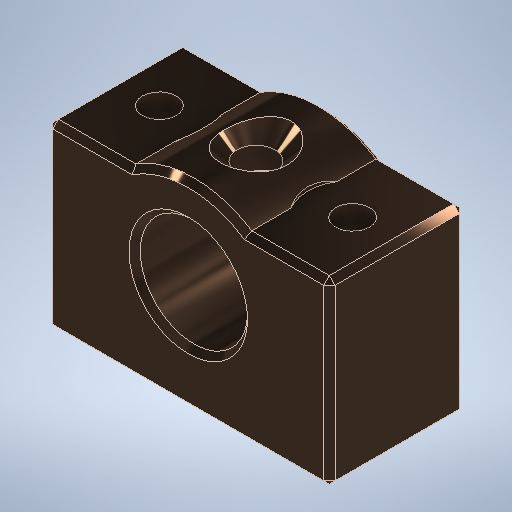
# Autodesk Inventor part: 05 Crankbearing
Saved by Autodesk Inventor 2025.2 (Build 292293000, 293)
## iProperties
Created: 2025-07-30
Part Number: 05 Crankbearing
Material: Bronze
Document SubType Name: Modeling
Designer: bless
Density: 8.47 g/cm^3
Appearance: Bronze - Polished
Author: bless
Autodesk Inventor part; units mm, degrees
ref_plane "YZ Plane" through (0, 0, 0) normal (1, 0, 0) x (0, 1, 0)
ref_plane "XY Plane" through (0, 0, 0) normal (0, 0, 1) x (1, 0, 0)
sketch "Sketch1" plane through (0, 0, 0) normal (0, 0, 1) x (1, 0, 0)
  line L0 (0, 0) -> (25, 0)
  line L1 (25, 0) -> (25, 16)
  line L2 (25, 16) -> (0, 16)
  line L3 (0, 16) -> (0, 0)
  circle A0 centre (12.5, 9.5) radius 4.75
  arc A1 (17.6235, 16) -> (7.3765, 16) centre (12.5, 8) ccw
  point P0 (12.5, 16)
  point P1 (0, 8)
  dimension "d0" = 25
  dimension "d1" = 16
  dimension "d2" = 9.5
  dimension "d6" = 9.5
  dimension "d7" = 9.5
  dimension "d8" = 7.3765
  dimension "d9" = 12.5
  constraints: 8 end point, 2 centre point, 2 midpoint, 2 parallel, 2 point on circle, 2 point on line, 1 horizontal, 1 perpendicular, 1 vertical alignment
  measures "d0" distance of L2.end L1.end
  measures "d1" distance of L1.end L0.end
  measures "d2" diameter of A0
  measures "d6" radius of A1
  measures "d7" distance from line of L0 A0.centre
  measures "d8" distance from line of A1.start L1
  measures "d9" distance from line of A1.centre L1
extrude "Extrusion1" add sketch "Sketch1" against normal blind 12
chamfer "Chamfer1" distance 0.5 angle 45 18 edges at (12.5, 17.5, 0) (3.6883, 16, 0) (21.3117, 16, 0) (25, 8, 0) (0, 8, 0) (25, 16, -6) (0, 16, -6) (21.3117, 16, -12) (12.5, 17.5, -12) (3.6883, 16, -12) (25, 8, -12) (0, 8, -12) (7.75, 9.5, 0) (7.75, 9.5, -12) (12.5, 0, 0) (25, 0, -6) (0, 0, -6) (12.5, 0, -12)
ref_plane "Work Plane1" through (0, 17.5, 0) normal (0, 1, 0) x (-1, 0, 0)
sketch "Sketch2" plane through (0, 17.5, 0) normal (0, 1, 0) x (-1, 0, 0)
  line L0 (-7.3765, -11.5) -> (-17.6235, -11.5) projected
  line L1 (-7.3765, -0.5) -> (-7.3765, -11.5) projected
  line L2 (-17.6235, -0.5) -> (-7.3765, -0.5) projected
  line L3 (-17.6235, -0.5) -> (-17.6235, -11.5) projected
  line L4 (-17.4749, -12) -> (-7.5251, -12) projected
  line L5 (-7.3765, -11.5) -> (-17.6235, -11.5) projected
  line L6 (-17.4749, 0) -> (-7.5251, 0) projected
  line L7 (-7.5251, 0) -> (-17.4749, 0) projected
  line L8 (-17.6235, -0.5) -> (-7.3765, -0.5) projected
  point P0 (0, 0)
  point P1 (-12.5, -6)
  point P2 (-12.5, -11.5)
  dimension "d16" = 5.5
  dimension "d17" = 5.1235
  constraints: 1 midpoint, 5 other
  measures "d16" distance of point (-12.5, -11.5) point (-12.5, -6)
  measures "d17" distance from line of L3 point (-12.5, -6)
hole "Hole1" at (12.5, 17.5, -6) direction (0, -1, 0) diameter 3.4 depth 9 countersink diameter 6.3 countersink angle 90
sketch "Sketch3" plane through (17.6235, 16, -11.5) normal (0, 1, 0) x (1, 0, 0)
  line L0 (6.8765, -11) -> (0, -11) projected
  line L1 (6.8765, 0) -> (6.8765, -11) projected
  circle A0 centre (3.4383, -5.5) radius 4
  line L2 (-17.1235, 0) -> (-10.247, 0) projected
  line L3 (-17.1235, -11) -> (-17.1235, 0) projected
  line L4 (-10.247, -11) -> (-17.1235, -11) projected
  line L5 (-10.247, -11) -> (-10.247, 0) projected
  circle A1 centre (-13.6852, -5.5) radius 4
  point P0 (-17.6235, -11.5)
  dimension "d25" = 4
  dimension "d26" = 4
  dimension "d27" = 3.4383
  dimension "d28" = 5.5
  dimension "d29" = 20.5617
  dimension "d30" = 5.5
  constraints: 2 centre point
  measures "d25" radius of A0
  measures "d26" radius of A1
  measures "d27" distance from line of A0.centre L1
  measures "d28" distance from line of A0.centre L0
  measures "d29" distance from line of A1.centre L1
  measures "d30" distance from line of A1.centre L0
extrude "Extrusion2" cut sketch "Sketch3" along normal through all contours A0 L1 | L1 A0 | A1 L5 L3 | L3 A1 | A1 L5
sketch "Sketch4" plane through (17.6235, 16, -11.5) normal (0, 1, 0) x (1, 0, 0)
  arc A0 (0, -3.4559) -> (0, -7.5441) centre (3.4383, -5.5) ccw projected
  line L0 (-10.247, -3.4559) -> (-10.247, 0) projected
  line L1 (-17.1235, 0) -> (-10.247, 0) projected
  line L2 (-17.1235, -11) -> (-17.1235, 0) projected
  line L3 (-10.247, -11) -> (-17.1235, -11) projected
  line L4 (-10.247, -11) -> (-10.247, -7.5441) projected
  arc A1 (-10.247, -7.5441) -> (-10.247, -3.4559) centre (-13.6852, -5.5) ccw projected
  point P0 (-17.6235, -11.5)
  constraints: 2 coincident
hole "Hole2" at (3.9383, 16, -6) at (21.0617, 16, -6) direction (0, -1, 0) diameter 3 end through all
body "Solid1"
